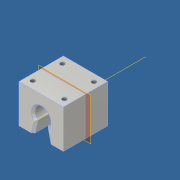
# Autodesk Inventor part: Linearwagen_20_kurz
Saved by Autodesk Inventor 2016 SP1 (Build 200210100, 210)
## iProperties
Created: 2016-01-01
Part Number: Linearwagen_20_kurz
Material: Aluminium 6061
Document SubType Name: Modeling
Designer: 4ndreas
Density: 2.7 g/cm^3
Appearance: Aluminium - flach
Mass: 69.857 g
Surface Area: 144.604 cm^2
Volume: 69.857 cm^3
Author: 4ndreas
Autodesk Inventor part; units mm, degrees
ref_plane "YZ Plane" through (0, 0, 0) normal (1, 0, 0) x (0, 1, 0)
ref_plane "XZ Plane" through (0, 0, 0) normal (0, 1, 0) x (-1, 0, 0)
ref_plane "XY Plane" through (0, 0, 0) normal (0, 0, 1) x (1, 0, 0)
sketch "Skizze1" plane through (0, 0, 0) normal (0, 0, 1) x (1, 0, 0)
  line L0 (-22.5, -22.5) -> (22.5, -22.5)
  line L1 (22.5, -22.5) -> (22.5, 22.5)
  line L2 (22.5, 22.5) -> (-22.5, 22.5)
  line L3 (-22.5, 22.5) -> (-22.5, -22.5)
  line L4 (-22.5, -22.5) -> (22.5, 22.5) construction
  line L5 (22.5, -22.5) -> (-22.5, 22.5) construction
  point P0 (0, 0)
  dimension "d0" = 45
  dimension "d1" = 45
  constraints: 12 end point, 2 midpoint, 2 parallel, 1 horizontal, 1 perpendicular
  measures "d0" distance between parallel lines of L0 L2
  measures "d1" distance between parallel lines of L1 L3
extrude "Extrusion1" add sketch "Skizze1" along normal blind 39
sketch "Skizze2" plane through (-22.5, -22.5, 0) normal (0, -1, 0) x (1, 0, 0)
  line L0 (0, 0) -> (45, 0) projected
  line L1 (45, 0) -> (45, 39) projected
  line L2 (0, 39) -> (45, 39) projected
  line L3 (0, 0) -> (0, 39) projected
  circle A0 centre (22.5, 19) radius 8
  line L4 (22.5, 0) -> (22.5, 39)
  line L5 (22.5, 19) -> (22.5, -6)
  line L6 (17.5, 12.755) -> (14.5, 0)
  line L7 (27.5, 12.755) -> (30.5, 0)
  dimension "d4" = 16
  dimension "d5" = 25
  dimension "d6" = 45
  dimension "d7" = 10
  dimension "d8" = 16
  constraints: 8 end point, 3 point on line, 2 point on circle, 1 centre point, 1 midpoint, 1 vertical, 1 other
  measures "d4" diameter of A0
  measures "d5" distance of L5.start L5.end
  measures "d6" distance from line of L5.end L2
  measures "d7" distance of L7.start L6.start
  measures "d8" distance of L7.end L6.end
extrude "Extrusion2" cut sketch "Skizze2" against normal through all contours L6 A0 L4 L0 | L4 A0 L7 L0 | A0 L4 | L4 A0
chamfer "Fase1" distance 2 angle 45 6 edges at (0, -22.5, 27) (-6.5, -22.5, 6.3775) (6.5, -22.5, 6.3775) (0, 22.5, 27) (-6.5, 22.5, 6.3775) (6.5, 22.5, 6.3775)
ref_plane "Arbeitsebene1" through (-22.5, 0, 39) normal (0, 1, 0) x (1, 0, 0)
sketch "Skizze3" plane through (0, 0, 39) normal (0, 0, 1) x (1, 0, 0)
  line L0 (-22.5, -22.5) -> (22.5, -22.5) projected
  line L1 (22.5, -22.5) -> (22.5, 22.5) projected
  line L2 (22.5, 22.5) -> (-22.5, 22.5) projected
  line L3 (-22.5, 22.5) -> (-22.5, -22.5) projected
  line L4 (16, -15) -> (-16, -15) construction
  line L5 (-16, -15) -> (-16, 15) construction
  line L6 (-16, 15) -> (16, 15) construction
  line L7 (16, 15) -> (16, -15) construction
  line L8 (16, -15) -> (-16, 15) construction
  line L9 (-16, -15) -> (16, 15) construction
  point P0 (0, 0)
  dimension "d14" = 32
  dimension "d15" = 30
  constraints: 12 end point, 2 midpoint, 2 parallel, 1 horizontal, 1 perpendicular
  measures "d14" distance between parallel lines of L7 L5
  measures "d15" distance between parallel lines of L6 L4
hole "Bohrung1" at (-16, -15, 39) at (16, -15, 39) at (-16, 15, 39) at (16, 15, 39) direction (0, 0, -1) diameter 4.134 depth 10 tip angle 118 thread size "M5x0.8" class "6H" standard "ANSI Metric M Profile"
